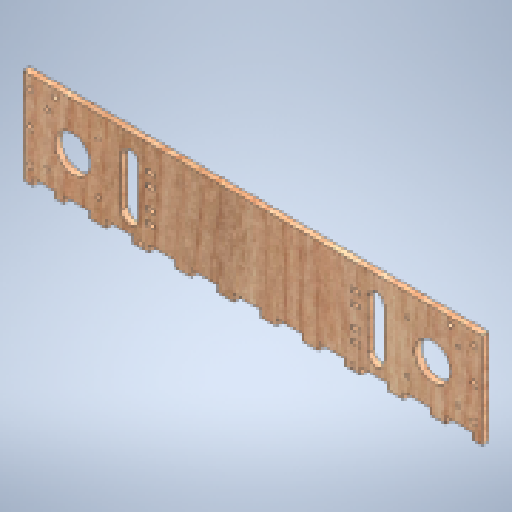
# Autodesk Inventor part: креп_мотора
Saved by Autodesk Inventor 2023.1 (Build 271208000, 208)
## iProperties
Created: 2025-12-22
Part Number: креп_мотора
Material: Древесина (береза)
Document SubType Name: Modeling
Designer: DELL
Density: 0.55 g/cm^3
Appearance: Береза — натуральный — полированный
Author: DELL
Autodesk Inventor part; units mm, degrees
ref_plane "YZ Plane" through (0, 0, 0) normal (1, 0, 0) x (0, 1, 0)
ref_plane "XZ Plane" through (0, 0, 0) normal (0, 1, 0) x (-1, 0, 0)
ref_plane "XY Plane" through (0, 0, 0) normal (0, 0, 1) x (1, 0, 0)
sketch "Эскиз1" plane through (0, 0, 0) normal (0, 0, 1) x (1, 0, 0)
  line L0 (-26.0621, -17.2379) -> (-22.2379, -21.0621) projected
  arc A0 (-22.2379, -21.0621) -> (-22.0257, -21.15) centre (-22.0257, -20.85) ccw projected
  line L1 (-22.0257, -21.15) -> (12.0257, -21.15) projected
  arc A1 (12.0257, -21.15) -> (12.2379, -21.0621) centre (12.0257, -20.85) ccw projected
  line L2 (12.2379, -21.0621) -> (16.0621, -17.2379) projected
  arc A2 (16.0621, -17.2379) -> (16.15, -17.0257) centre (15.85, -17.0257) ccw projected
  line L3 (16.15, -17.0257) -> (16.15, 17.0257) projected
  arc A3 (16.15, 17.0257) -> (16.0621, 17.2379) centre (15.85, 17.0257) ccw projected
  line L4 (16.0621, 17.2379) -> (12.2379, 21.0621) projected
  arc A4 (12.2379, 21.0621) -> (12.0257, 21.15) centre (12.0257, 20.85) ccw projected
  line L5 (12.0257, 21.15) -> (-22.0257, 21.15) projected
  arc A5 (-22.0257, 21.15) -> (-22.2379, 21.0621) centre (-22.0257, 20.85) ccw projected
  line L6 (-22.2379, 21.0621) -> (-26.0621, 17.2379) projected
  arc A6 (-26.0621, 17.2379) -> (-26.15, 17.0257) centre (-25.85, 17.0257) ccw projected
  line L7 (-26.15, 17.0257) -> (-26.15, -17.0257) projected
  arc A7 (-26.15, -17.0257) -> (-26.0621, -17.2379) centre (-25.85, -17.0257) ccw projected
  circle A8 centre (-5, 0) radius 11 projected
  circle A9 centre (-20.5, 15.5) radius 1.25 projected
  circle A10 centre (10.5, 15.5) radius 1.25 projected
  circle A11 centre (10.5, -15.5) radius 1.25 projected
  circle A12 centre (-20.5, -15.5) radius 1.25 projected
  circle A13 centre (20.65, -19.15) radius 1.75 projected
  circle A14 centre (20.65, 0.85) radius 1.75 projected
  circle A15 centre (20.65, 20.85) radius 1.75 projected
  circle A16 centre (20.65, 40.85) radius 1.75 projected
  line L8 (-246.5621, -17.2379) -> (-242.7379, -21.0621) projected
  arc A17 (-242.7379, -21.0621) -> (-242.5257, -21.15) centre (-242.5257, -20.85) ccw projected
  line L9 (-242.5257, -21.15) -> (-208.4743, -21.15) projected
  arc A18 (-208.4743, -21.15) -> (-208.2621, -21.0621) centre (-208.4743, -20.85) ccw projected
  line L10 (-208.2621, -21.0621) -> (-204.4379, -17.2379) projected
  arc A19 (-204.4379, -17.2379) -> (-204.35, -17.0257) centre (-204.65, -17.0257) ccw projected
  line L11 (-204.35, -17.0257) -> (-204.35, 17.0257) projected
  arc A20 (-204.35, 17.0257) -> (-204.4379, 17.2379) centre (-204.65, 17.0257) ccw projected
  line L12 (-204.4379, 17.2379) -> (-208.2621, 21.0621) projected
  arc A21 (-208.2621, 21.0621) -> (-208.4743, 21.15) centre (-208.4743, 20.85) ccw projected
  line L13 (-208.4743, 21.15) -> (-242.5257, 21.15) projected
  arc A22 (-242.5257, 21.15) -> (-242.7379, 21.0621) centre (-242.5257, 20.85) ccw projected
  line L14 (-242.7379, 21.0621) -> (-246.5621, 17.2379) projected
  arc A23 (-246.5621, 17.2379) -> (-246.65, 17.0257) centre (-246.35, 17.0257) ccw projected
  line L15 (-246.65, 17.0257) -> (-246.65, -17.0257) projected
  arc A24 (-246.65, -17.0257) -> (-246.5621, -17.2379) centre (-246.35, -17.0257) ccw projected
  circle A25 centre (-225.5, 0) radius 11 projected
  circle A26 centre (-241, 15.5) radius 1.25 projected
  circle A27 centre (-210, 15.5) radius 1.25 projected
  circle A28 centre (-210, -15.5) radius 1.25 projected
  circle A29 centre (-241, -15.5) radius 1.25 projected
  circle A30 centre (-251.15, -19.15) radius 1.75 projected
  circle A31 centre (-251.15, 0.85) radius 1.75 projected
  circle A32 centre (-251.15, 20.85) radius 1.75 projected
  circle A33 centre (-251.15, 40.85) radius 1.75 projected
  line L16 (-255.45, -29.15) -> (-246.85, -29.15) projected
  line L17 (-255.65, -29.15) -> (-255.65, 270.85) projected
  line L18 (25.15, 270.85) -> (25.15, -29.15) projected
  line L19 (25.15, -29.15) -> (-255.65, -29.15)
  line L20 (-255.65, -29.15) -> (-255.65, 45.35)
  line L21 (25.15, 45.35) -> (25.15, -29.15)
  line L22 (25.15, 28.85) -> (-255.65, 28.85)
  dimension "d63" = 58
  constraints: 8 end point, 3 point on line, 2 perpendicular, 1 horizontal, 1 parallel
  measures "d63" distance between parallel lines of L22 L19
extrude "Выдавливание1" add sketch "Эскиз1" along normal blind 4 contours A7 L7 A6 L6 A5 L5 A4 L4 A3 L3 A2 L2 A1 L1 A0 L0 | A24 L15 A23 L14 A22 L13 A21 L12 A20 L11 A19 L10 A18 L9 A17 L8 | L19 L17 L22 L18 L16
sketch "Эскиз2" plane through (0, 0, 4) normal (0, 0, 1) x (1, 0, 0)
  circle A0 centre (5.65, 24.85) radius 1.6
  circle A1 centre (-236.15, 24.85) radius 1.6
  circle A2 centre (20.65, 20.85) radius 1.75 construction
  line L0 (20.65, 20.85) -> (-7.9342, 20.85) construction
  circle A3 centre (-251.15, 20.85) radius 1.75 construction
  circle A4 centre (-251.15, 20.85) radius 1.75 construction
  line L1 (-251.15, 20.85) -> (-207.2743, 20.85) construction
  line L2 (20.65, 20.85) -> (20.65, 34.2007) construction
  point P0 (0, 0)
  point P1 (20.65, 40.85)
  dimension "d16" = 3.2
  dimension "d18" = 3.2
  dimension "d93" = 15
  dimension "d94" = 4
  dimension "d104" = 4
  dimension "d105" = 15
  constraints: 6 end point, 2 centre point, 2 horizontal, 1 vertical
  measures "d16" diameter of A0
  measures "d18" diameter of A1
  measures "d93" distance from line of A0.centre L2
  measures "d94" distance from line of L0 A0.centre
  measures "d104" distance from line of L1 A1.centre
  measures "d105" horizontal distance of A3.centre A1.centre
extrude "Выдавливание2" cut sketch "Эскиз2" against normal blind 6
sketch "Эскиз7" plane through (0, 0, 0) normal (0, 0, -1) x (-1, 0, 0)
  line L0 (-25.15, -29.15) -> (-25.15, 28.85) projected
  line L1 (-25.15, -0.15) -> (255.65, -0.15) construction
  line L2 (255.65, 28.85) -> (255.65, -29.15) projected
  line L3 (190.65, -15.15) -> (190.65, 14.85) construction
  line L4 (195.65, -15.15) -> (195.65, 14.85)
  line L5 (185.65, 14.85) -> (185.65, -15.15)
  arc A0 (185.65, -15.15) -> (195.65, -15.15) centre (190.65, -15.15) ccw
  arc A1 (195.65, 14.85) -> (185.65, 14.85) centre (190.65, 14.85) ccw
  line L6 (115.25, -0.15) -> (115.25, 45.35) construction
  line L7 (39.85, -15.15) -> (39.85, 14.85) construction
  line L8 (34.85, -15.15) -> (34.85, 14.85)
  line L9 (44.85, 14.85) -> (44.85, -15.15)
  arc A2 (34.85, -15.15) -> (44.85, -15.15) centre (39.85, -15.15) ccw
  arc A3 (44.85, 14.85) -> (34.85, 14.85) centre (39.85, 14.85) ccw
  point P0 (0, 0)
  point P1 (-25.15, 45.35)
  point P2 (255.65, 45.35)
  point P3 (190.65, -0.15)
  point P4 (39.85, -0.15)
  dimension "d56" = 15
  dimension "d57" = 10
  dimension "d58" = 60
  constraints: 20 end point, 8 point on circle, 7 symmetric about line, 4 centre point, 4 midpoint, 4 tangent, 1 parallel, 1 perpendicular, 1 point on line, 1 vertical, 2 other
  measures "d56" distance of point (190.65, -0.15) L3.end
  measures "d57" diameter of A1
  measures "d58" distance between parallel lines of L2 L4
extrude "Выдавливание7" cut sketch "Эскиз7" against normal blind 10
sketch "Эскиз8" plane through (0, 0, 4) normal (0, 0, 1) x (1, 0, 0)
  line L0 (-255.65, -29.15) -> (25.15, -29.15) projected
  line L1 (19.15, -29.15) -> (3.15, -29.15)
  line L2 (3.15, -29.15) -> (3.15, -25.15)
  line L3 (3.15, -25.15) -> (19.15, -25.15)
  line L4 (19.15, -25.15) -> (19.15, -29.15)
  line L5 (25.15, -29.15) -> (25.15, 28.85) projected
  line L6 (-22.85, -25.15) -> (-6.85, -25.15)
  line L7 (-22.85, -29.15) -> (-22.85, -25.15)
  line L8 (-6.85, -29.15) -> (-22.85, -29.15)
  line L9 (-6.85, -25.15) -> (-6.85, -29.15)
  line L10 (-48.85, -25.15) -> (-32.85, -25.15)
  line L11 (-48.85, -29.15) -> (-48.85, -25.15)
  line L12 (-32.85, -29.15) -> (-48.85, -29.15)
  line L13 (-32.85, -25.15) -> (-32.85, -29.15)
  line L14 (-74.85, -25.15) -> (-58.85, -25.15)
  line L15 (-74.85, -29.15) -> (-74.85, -25.15)
  line L16 (-58.85, -29.15) -> (-74.85, -29.15)
  line L17 (-58.85, -25.15) -> (-58.85, -29.15)
  line L18 (-100.85, -25.15) -> (-84.85, -25.15)
  line L19 (-100.85, -29.15) -> (-100.85, -25.15)
  line L20 (-84.85, -29.15) -> (-100.85, -29.15)
  line L21 (-84.85, -25.15) -> (-84.85, -29.15)
  line L22 (-126.85, -25.15) -> (-110.85, -25.15)
  line L23 (-126.85, -29.15) -> (-126.85, -25.15)
  line L24 (-110.85, -29.15) -> (-126.85, -29.15)
  line L25 (-110.85, -25.15) -> (-110.85, -29.15)
  line L26 (-152.85, -25.15) -> (-136.85, -25.15)
  line L27 (-152.85, -29.15) -> (-152.85, -25.15)
  line L28 (-136.85, -29.15) -> (-152.85, -29.15)
  line L29 (-136.85, -25.15) -> (-136.85, -29.15)
  line L30 (-178.85, -25.15) -> (-162.85, -25.15)
  line L31 (-178.85, -29.15) -> (-178.85, -25.15)
  line L32 (-162.85, -29.15) -> (-178.85, -29.15)
  line L33 (-162.85, -25.15) -> (-162.85, -29.15)
  line L34 (-204.85, -25.15) -> (-188.85, -25.15)
  line L35 (-204.85, -29.15) -> (-204.85, -25.15)
  line L36 (-188.85, -29.15) -> (-204.85, -29.15)
  line L37 (-188.85, -25.15) -> (-188.85, -29.15)
  line L38 (-230.85, -25.15) -> (-214.85, -25.15)
  line L39 (-230.85, -29.15) -> (-230.85, -25.15)
  line L40 (-214.85, -29.15) -> (-230.85, -29.15)
  line L41 (-214.85, -25.15) -> (-214.85, -29.15)
  line L42 (-255.65, -29.15) -> (25.15, -29.15) projected
  line L43 (-236.85, -29.15) -> (-249.65, -29.15)
  line L44 (-249.65, -29.15) -> (-249.65, -25.15)
  line L45 (-249.65, -25.15) -> (-236.85, -25.15)
  line L46 (-236.85, -25.15) -> (-236.85, -29.15)
  line L47 (-255.65, 28.85) -> (-255.65, -29.15) projected
  point P0 (-249.65, -29.15)
  point P1 (-152.85, -29.15)
  point P2 (-136.85, -29.15)
  point P3 (-178.85, -29.15)
  point P4 (-162.85, -29.15)
  point P5 (-204.85, -29.15)
  point P6 (-188.85, -29.15)
  point P7 (-230.85, -29.15)
  point P8 (-214.85, -29.15)
  point P9 (-126.85, -29.15)
  point P10 (-110.85, -29.15)
  point P11 (-100.85, -29.15)
  point P12 (-84.85, -29.15)
  point P13 (-74.85, -29.15)
  point P14 (-58.85, -29.15)
  point P15 (-48.85, -29.15)
  point P16 (-32.85, -29.15)
  point P17 (-22.85, -29.15)
  dimension "d75" = 16
  dimension "d76" = 4
  dimension "d77" = 6
  dimension "d80" = 26
  dimension "d86" = 4
  dimension "d87" = 6
  dimension "d88" = 6
  constraints: 88 end point, 36 horizontal alignment, 22 parallel, 18 collinear, 2 horizontal, 2 perpendicular, 4 other
  measures "d75" distance of L2.end L3.end
  measures "d76" distance of L1.end L2.end
  measures "d77" distance between parallel lines of L5 L4
  measures "d80" distance of L2.end L6.start
  measures "d86" distance of L43.end L44.end
  measures "d87" distance between parallel lines of L47 L44
  measures "d88" distance between parallel lines of L39 L46
extrude "Выдавливание8" cut sketch "Эскиз8" against normal blind 4
sketch "Эскиз9" plane through (0, 0, 0) normal (0, 0, -1) x (-1, 0, 0)
  line L0 (48.85, -25.15) -> (48.85, -29.15) construction
  line L1 (58.85, -25.15) -> (48.85, -29.15) construction
  line L2 (188.85, -29.15) -> (188.85, -25.15) construction
  line L3 (178.85, -25.15) -> (178.85, -29.15) construction
  line L4 (188.85, -25.15) -> (178.85, -29.15) construction
  circle A0 centre (183.85, -27.15) radius 1.65
  circle A1 centre (53.85, -27.15) radius 1.65
  point P0 (0, 0)
  dimension "d89" = 3.3
  dimension "d90" = 3.3
  constraints: 4 end point, 2 centre point, 2 midpoint
  measures "d89" diameter of A0
  measures "d90" diameter of A1
extrude "Выдавливание9" cut sketch "Эскиз9" against normal blind 4
sketch "Эскиз10" plane through (0, 0, 0) normal (0, 0, -1) x (-1, 0, 0)
  line L0 (49.85, -15.15) -> (54.85, -15.15)
  line L1 (54.85, -15.15) -> (54.85, -12.65)
  line L2 (54.85, -12.65) -> (49.85, -12.65)
  line L3 (49.85, -12.65) -> (49.85, -15.15)
  line L4 (49.85, -7.65) -> (54.85, -7.65)
  line L5 (54.85, -7.65) -> (54.85, -5.15)
  line L6 (54.85, -5.15) -> (49.85, -5.15)
  line L7 (49.85, -5.15) -> (49.85, -7.65)
  line L8 (44.85, -15.15) -> (44.85, 14.85) construction
  line L9 (44.85, -0.15) -> (59.3137, -0.15) construction
  line L10 (49.85, 14.85) -> (54.85, 14.85)
  line L11 (54.85, 14.85) -> (54.85, 12.35)
  line L12 (54.85, 12.35) -> (49.85, 12.35)
  line L13 (49.85, 12.35) -> (49.85, 14.85)
  line L14 (49.85, 7.35) -> (54.85, 7.35)
  line L15 (54.85, 7.35) -> (54.85, 4.85)
  line L16 (54.85, 4.85) -> (49.85, 4.85)
  line L17 (49.85, 4.85) -> (49.85, 7.35)
  line L18 (-25.15, 28.85) -> (255.65, 28.85) projected
  line L19 (115.25, 28.85) -> (115.25, -15.15) construction
  line L20 (180.65, -15.15) -> (175.65, -15.15)
  line L21 (175.65, -15.15) -> (175.65, -12.65)
  line L22 (175.65, -12.65) -> (180.65, -12.65)
  line L23 (180.65, -12.65) -> (180.65, -15.15)
  line L24 (180.65, -7.65) -> (175.65, -7.65)
  line L25 (175.65, -7.65) -> (175.65, -5.15)
  line L26 (175.65, -5.15) -> (180.65, -5.15)
  line L27 (180.65, -5.15) -> (180.65, -7.65)
  line L28 (185.65, -0.15) -> (171.1863, -0.15) construction
  line L29 (180.65, 14.85) -> (175.65, 14.85)
  line L30 (175.65, 14.85) -> (175.65, 12.35)
  line L31 (175.65, 12.35) -> (180.65, 12.35)
  line L32 (180.65, 12.35) -> (180.65, 14.85)
  line L33 (180.65, 7.35) -> (175.65, 7.35)
  line L34 (175.65, 7.35) -> (175.65, 4.85)
  line L35 (175.65, 4.85) -> (180.65, 4.85)
  line L36 (180.65, 4.85) -> (180.65, 7.35)
  point P0 (0, 0)
  dimension "d95" = 5
  dimension "d96" = 2.5
  dimension "d97" = 5
  dimension "d98" = 2.5
  dimension "d99" = 5
  dimension "d102" = 5
  dimension "d103" = 5
  constraints: 70 end point, 26 symmetric about line, 4 parallel, 3 horizontal, 2 midpoint, 2 perpendicular, 1 vertical
  measures "d95" distance of L2.end L1.end
  measures "d96" distance of L1.end L0.end
  measures "d97" distance of L6.end L5.end
  measures "d98" distance of L5.end L4.end
  measures "d99" distance between parallel lines of L4 L2
  measures "d102" distance between parallel lines of L8 L3
  measures "d103" distance between parallel lines of L8 L7
extrude "Выдавливание10" cut sketch "Эскиз10" against normal blind 10
